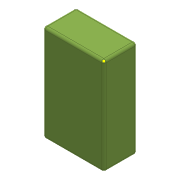
# Autodesk Inventor part: BatteryBox
Saved by Autodesk Inventor 2018 (Build 220112000, 112)
## iProperties
Created: 2018-09-24
Part Number: BatteryBox
Material: Generic
Document SubType Name: Modeling
Designer: DCCUMD
Density: 1 g/cm^3
Appearance: Olive Green
Author: DCCUMD
Autodesk Inventor part; units mm, degrees
ref_plane "YZ Plane" through (0, 0, 0) normal (1, 0, 0) x (0, 1, 0)
ref_plane "XZ Plane" through (0, 0, 0) normal (0, 1, 0) x (-1, 0, 0)
ref_plane "XY Plane" through (0, 0, 0) normal (0, 0, 1) x (1, 0, 0)
sketch "Sketch1" plane through (0, 0, 0) normal (0, 1, 0) x (-1, 0, 0)
  line L0 (0, 0) -> (48.8, 0)
  line L1 (48.8, 0) -> (48.8, -77.5)
  line L2 (48.8, -77.5) -> (0, -77.5)
  line L3 (0, -77.5) -> (0, 0)
  dimension "d0" = 48.8
  dimension "d1" = 77.5
  constraints: 8 end point, 2 parallel, 1 horizontal, 1 perpendicular
  measures "d0" distance of L1.end L2.end
  measures "d1" distance between parallel lines of L2 L0
extrude "Extrusion1" add sketch "Sketch1" along normal blind 26.7
fillet "Fillet1" radius 2 12 edges at (0, 13.35, 0) (-48.8, 13.35, 0) (-48.8, 26.7, -38.75) (0, 26.7, -38.75) (-24.4, 26.7, 0) (-24.4, 26.7, -77.5) (-24.4, 0, -77.5) (-48.8, 13.35, -77.5) (-48.8, 0, -38.75) (-24.4, 0, 0) (0, 0, -38.75) (0, 13.35, -77.5)
sketch "Sketch2" plane through (0, 0, 0) normal (0, -1, 0) x (1, 0, 0)
  point P0 (0, 0)
body "Solid1"
